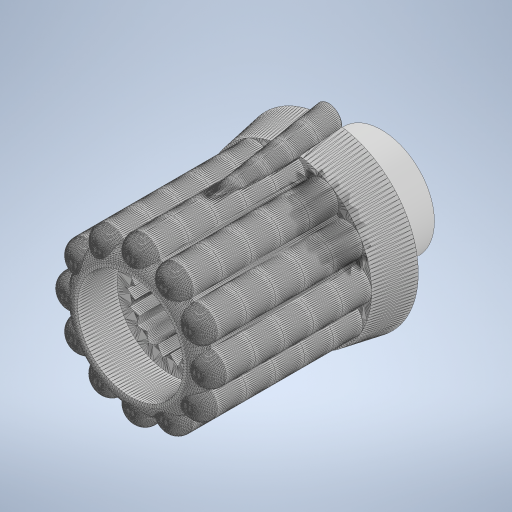
# Autodesk Inventor part: Volume_Cnob4
Saved by Autodesk Inventor 2024 (Build 280153000, 153)
## iProperties
Created: 2023-06-19
Part Number: Volume_Cnob4
Material: Типовые
Document SubType Name: Modeling
Designer: fm
Density: 1 g/cm^3
Appearance: По умолчанию
Author: fm
Autodesk Inventor part; units mm, degrees
ref_plane "YZ Plane" through (0, 0, 0) normal (1, 0, 0) x (0, 1, 0)
ref_plane "XZ Plane" through (0, 0, 0) normal (0, 1, 0) x (-1, 0, 0)
ref_plane "XY Plane" through (0, 0, 0) normal (0, 0, 1) x (1, 0, 0)
sketch "Эскиз1" plane through (-0.5591, 3.1708, 0) normal (0, 0, -1) x (-1, 0, 0)
  circle A0 centre (-0.5585, -3.1706) radius 6.7783
  arc A1 (0.4399, 3.5338) -> (-1.5581, 3.5336) centre (-0.5591, 3.5791) ccw
  arc A2 (0.3612, -0.6338) -> (-0.0025, -0.0021) centre (-1.4904, -1.2792) ccw
  arc A3 (-0.562, -0.4721) -> (-1.1198, -0.0028) centre (-2.0812, -1.7119) ccw
  arc A4 (-0.0025, -0.0021) -> (-0.562, -0.4721) centre (1.1062, -1.8903) ccw
  arc A5 (1.0485, -0.3834) -> (0.3612, -0.6338) centre (1.4437, -2.537) ccw
  arc A6 (1.1741, -1.1052) -> (1.0485, -0.3834) centre (-0.7873, -1.0749) ccw
  arc A7 (1.9074, -1.1012) -> (1.1741, -1.1052) centre (1.5506, -2.9063) ccw
  arc A8 (3.4203, -2.9369) -> (3.4202, -2.9367) centre (1.5368, -3.3481) ccw
  arc A9 (2.4636, -4.2712) -> (2.0999, -3.6397) centre (0.4108, -5.0328) ccw
  arc A10 (2.4603, -2.0702) -> (1.7761, -1.8226) centre (1.4734, -3.7283) ccw
  arc A11 (2.399, -2.2239) -> (2.3988, -2.2237) centre (1.3794, -3.9805) ccw
  arc A12 (2.6578, -3.1705) -> (2.0967, -2.6994) centre (0.989, -4.5881) ccw
  arc A13 (1.7048, -3.2697) -> (1.704, -3.2691) centre (0.4108, -5.0328) ccw
  arc A14 (2.1142, -1.9099) -> (2.1147, -1.9084) centre (-0.0255, -1.1393) ccw
  arc A15 (2.0967, -2.6994) -> (2.4603, -2.0702) centre (0.6102, -1.4206) ccw
  arc A16 (1.7761, -1.8226) -> (1.9074, -1.1012) centre (-0.0212, -1.1229) ccw
  arc A17 (2.0999, -3.6397) -> (2.6578, -3.1705) centre (0.9892, -1.753) ccw
  arc A18 (1.7732, -4.5186) -> (2.4636, -4.2712) centre (1.4494, -2.5283) ccw
  arc A19 (-2.2398, 0.2426) -> (-2.2407, 0.2425) centre (-2.0812, -1.7119) ccw
  arc A20 (-2.6567, 0.1627) -> (-2.657, 0.1626) centre (-2.0812, -1.7119) ccw
  arc A21 (-1.1198, -0.0028) -> (-1.4869, -0.6353) centre (0.5636, -1.4028) ccw
  arc A22 (-2.1711, -0.3856) -> (-2.2993, -1.1005) centre (-0.0255, -1.1393) ccw
  arc A23 (-2.2993, -1.1005) -> (-3.0268, -1.1018) centre (-2.6591, -3.2603) ccw
  arc A24 (-3.0268, -1.1018) -> (-2.9013, -1.8244) centre (-0.7528, -1.0789) ccw
  arc A25 (-1.4869, -0.6353) -> (-2.1711, -0.3856) centre (-2.4895, -2.3203) ccw
  arc A26 (-3.5831, -0.465) -> (-3.5898, -0.4828) centre (-1.456, -1.2707) ccw
  arc A27 (-3.5856, -2.0697) -> (-3.2205, -2.706) centre (-1.456, -1.2707) ccw
  arc A28 (-3.5481, -0.4455) -> (-3.5831, -0.465) centre (-2.5019, -2.3689) ccw
  arc A29 (-3.5481, -0.4455) -> (-3.5898, -0.4828) centre (-2.2613, -1.9251) ccw
  arc A30 (-2.9034, -1.8182) -> (-3.5856, -2.0697) centre (-2.468, -4.0503) ccw
  arc A31 (-3.2205, -2.706) -> (-3.7771, -3.1692) centre (-2.23, -4.4624) ccw
  arc A32 (-3.2141, -3.6391) -> (-3.5821, -4.2735) centre (-1.7608, -4.9061) ccw
  arc A33 (-3.7771, -3.1692) -> (-3.2141, -3.6391) centre (-2.2613, -1.9251) ccw
  arc A34 (-3.5821, -4.2735) -> (-2.8961, -4.5227) centre (-2.5019, -2.3689) ccw
  arc A35 (-2.8961, -4.5227) -> (-3.0256, -5.2404) centre (-1.0091, -5.2336) ccw
  arc A36 (-3.0256, -5.2404) -> (-2.2923, -5.2364) centre (-2.6703, -3.165) ccw
  arc A37 (-2.2923, -5.2364) -> (-2.169, -5.9592) centre (0.1297, -5.1949) ccw
  arc A38 (-2.169, -5.9592) -> (-1.4813, -5.7046) centre (-2.4696, -4.0912) ccw
  arc A39 (-1.4813, -5.7046) -> (-1.1182, -6.3416) centre (0.415, -5.0456) ccw
  arc A40 (-1.1182, -6.3416) -> (-0.5591, -5.8672) centre (-2.1317, -4.5805) ccw
  arc A41 (-0.5591, -5.8672) -> (0, -6.3416) centre (0.9916, -4.6063) ccw
  arc A42 (0, -6.3416) -> (0.3631, -5.7046) centre (-1.6247, -4.9934) ccw
  arc A43 (0.3631, -5.7046) -> (1.0508, -5.9592) centre (1.3221, -4.1702) ccw
  arc A44 (1.0508, -5.9592) -> (1.1741, -5.2364) centre (-0.8689, -5.2596) ccw
  arc A45 (1.1741, -5.2364) -> (1.9074, -5.2404) centre (1.5505, -3.4608) ccw
  arc A46 (1.9074, -5.2404) -> (1.7732, -4.5186) centre (0.0238, -5.217) ccw
  circle A47 centre (-0.5585, -3.1706) radius 4
  point P0 (-2.8943, -1.8226)
  point P1 (-3.0256, -1.1012)
  point P2 (-2.2923, -1.1052)
  point P3 (-2.169, -0.3824)
  point P4 (-1.4813, -0.637)
  point P5 (-1.1182, 0)
  point P6 (-0.5591, -0.4744)
  point P7 (0, 0)
  point P8 (0.3631, -0.637)
  point P9 (1.0508, -0.3824)
  point P10 (2.4665, -2.0696)
  point P11 (2.0964, -2.7026)
  point P12 (2.6606, -3.1708)
  point P13 (2.0964, -3.639)
  point P14 (2.4665, -4.272)
  point P15 (1.7761, -4.519)
  point P16 (-3.0256, -5.2404)
  point P17 (-2.8943, -4.519)
  point P18 (-3.5847, -4.272)
  point P19 (-3.2146, -3.639)
  point P20 (-3.7788, -3.1708)
  point P21 (-3.2146, -2.7026)
  point P22 (-3.5847, -2.0696)
  dimension "d0" = 8
  constraints: 99 point on circle, 48 centre point, 4 coincident
  measures "d0" diameter of A47
extrude "Выдавливание1" add sketch "Эскиз1" along normal blind 4 contours A2 A4 A3 A19 A14 A47 A8 A16 A7 A6 A5 | A21 A25 A14 A19 | A19 A47 A14 | A14 A23 A24 A30 A27 A31 A19 A47 | A8 A14 A10 A16 | A31 A33 A32 A34 A35 A36 A37 A38 A13 A47 A19 | A14 A47 A8 | A8 A47 A11 A15 A10 A14 | A38 A39 A40 A41 A42 A11 A13 A47 | A42 A43 A44 A8 A13 A11 | A11 A47 A8 A13 A9 A17 A12 A15 | A13 A11 A47 | A13 A8 A47 A11 | A13 A8 A46 A18
